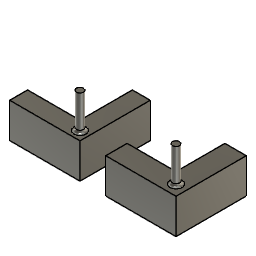
Laser+L_s (Autodesk Fusion 360 design; units mm, degrees)
Autodesk Fusion 360 part; units mm, degrees
note: some values were not read from the file. Set by a fixed rule: which sketch regions a step uses.
sketch "Sketch1" plane through (0, 0, 0) normal (0, 0, 1) x (1, 0, 0)
  line L0 (0, 0) -> (20.5, 0)
  line L1 (20.5, 0) -> (20.5, 80.5)
  line L2 (20.5, 80.5) -> (0, 80.5)
  line L3 (0, 80.5) -> (0, 0)
  line L4 (0, 0) -> (-60, 0)
  line L5 (-60, 0) -> (-60, 20.5)
  line L6 (-60, 20.5) -> (0, 20.5)
  line L7 (0, 20.5) -> (0, 0)
  dimension "d1" = 20.5
  dimension "d2" = 60
  dimension "d3" = 20.5
  dimension "d4" = 80.5
  constraint horizontal L0
  constraint vertical L1
  constraint horizontal L2
  constraint vertical L3
  constraint coincident L0.start L3.end
  constraint horizontal L4
  constraint vertical L5
  constraint horizontal L6
  constraint vertical L7
  measures "d1" distance of L0.start L0.end
  measures "d2" distance of L5.end L6.end
  measures "d3" distance of L4.end L5.end
  measures "d4" distance of L0.end L1.end
extrude "Extrude1" add sketch "Sketch1" along normal blind 40 makes body 1
sketch "Sketch3" plane through (0, 0, 0) normal (0, 0, -1) x (1, 0, 0)
  line L0 (20.5, 0) -> (-60, 0)
  line L1 (-60, 0) -> (-60, -20.5)
  line L2 (-60, -20.5) -> (0, -20.5)
  line L3 (0, -20.5) -> (0, -80.5)
  line L4 (0, -80.5) -> (20.5, -80.5)
  line L5 (20.5, -80.5) -> (20.5, 0)
  line L6 (14.0377, -6.3471) -> (0.9042, -6.3471) construction
  line L7 (0.9042, -6.3471) -> (0.9042, -16.8864) construction
  line L8 (0.9042, -16.8864) -> (14.0377, -16.8864) construction
  line L9 (14.0377, -16.8864) -> (14.0377, -6.3471) construction
  dimension "d7" = 12
  text T0 "R" font "Arial" height 12 align left top in box 13.1336 x 10.5393 at (14.0377, -6.3471) x (-1, 0) y (0, -1) spacing 1
extrude "Extrude2" cut sketch "Sketch3" against normal blind 3 text T0 bodies 1
sketch "Sketch4" plane through (0, 0, 40) normal (0, 0, 1) x (-1, 0, 0)
  line L0 (60, 0) -> (-20.5, 0)
  line L1 (-20.5, 0) -> (-20.5, -80.5)
  line L2 (-20.5, -80.5) -> (0, -80.5)
  line L3 (0, -80.5) -> (0, -20.5)
  line L4 (0, -20.5) -> (60, -20.5)
  line L5 (60, -20.5) -> (60, 0)
  line L6 (0, -20.5) -> (-20.5, 0)
  circle A0 centre (-10.25, -10.25) radius 4
  dimension "d10" = 8
  constraint coincident L3.end L4.start
  constraint coincident L0.end L1.start
  constraint midpoint L6 A0.centre
  measures "d10" diameter of A0
extrude "Extrude3" add sketch "Sketch4" along normal blind 40 contours L6 A0 | L6 A0 bodies 1
fillet "Fillet1" radius 3 1 edges at (13.9793, 8.8035, 40) on bodies 1
sketch "Sketch5" plane through (0, 0, 0) normal (0, 0, 1) x (1, 0, 0)
  line L0 (50, 0) -> (130.5, 0)
  line L1 (130.5, 0) -> (130.5, 24.5)
  line L2 (130.5, 24.5) -> (50, 24.5)
  line L3 (50, 24.5) -> (50, 0)
  line L4 (130.5, 0) -> (106, 0)
  line L5 (106, 0) -> (106, 80.5)
  line L6 (106, 80.5) -> (130.5, 80.5)
  line L7 (130.5, 80.5) -> (130.5, 0)
  dimension "d15" = 24.5
  dimension "d16" = 80.5
  dimension "d17" = 24.5
  dimension "d18" = 80.5
  constraint horizontal L0
  constraint vertical L1
  constraint horizontal L2
  constraint vertical L3
  constraint horizontal L4
  constraint vertical L5
  constraint horizontal L6
  constraint vertical L7
  measures "d15" distance of L0.start L2.end
  measures "d16" distance of L0.start L0.end
  measures "d17" distance of L0.end L4.end
  measures "d18" distance of L0.end L6.end
extrude "Extrude4" add sketch "Sketch5" along normal blind 40 separate body makes body 2
sketch "Sketch6" plane through (0, 0, 0) normal (0, 0, -1) x (1, 0, 0)
  line L0 (50, -24.5) -> (106, -24.5)
  line L1 (106, -24.5) -> (106, -80.5)
  line L2 (106, -80.5) -> (130.5, -80.5)
  line L3 (130.5, -80.5) -> (130.5, 0)
  line L4 (130.5, 0) -> (50, 0)
  line L5 (50, 0) -> (50, -24.5)
  line L6 (120.6614, -6.2816) -> (105.6614, -6.2816) construction
  line L7 (105.6614, -6.2816) -> (105.6614, -21.2816) construction
  line L8 (105.6614, -21.2816) -> (120.6614, -21.2816) construction
  line L9 (120.6614, -21.2816) -> (120.6614, -6.2816) construction
  dimension "d21" = 12
  text T0 "L" font "Arial" height 12 align left top in box 15 x 15 at (120.6614, -6.2816) x (-1, 0) y (0, -1) spacing 1
extrude "Extrude5" cut sketch "Sketch6" against normal blind 3 text T0 bodies 2
sketch "Sketch7" plane through (0, 0, 40) normal (0, 0, 1) x (-1, 0, 0)
  line L0 (-106, -24.5) -> (-50, -24.5)
  line L1 (-50, -24.5) -> (-50, 0)
  line L2 (-50, 0) -> (-130.5, 0)
  line L3 (-130.5, 0) -> (-130.5, -80.5)
  line L4 (-130.5, -80.5) -> (-106, -80.5)
  line L5 (-106, -80.5) -> (-106, -24.5)
  line L6 (-106, -24.5) -> (-130.5, 0)
  circle A0 centre (-118.25, -12.25) radius 4
  dimension "d24" = 8
  constraint coincident L0.start L5.end
  constraint coincident L2.end L3.start
  constraint midpoint L6 A0.centre
  measures "d24" diameter of A0
extrude "Extrude6" add sketch "Sketch7" along normal blind 40 contours L6 A0 | L6 A0 bodies 2
fillet "Fillet2" radius 3 1 edges at (121.9793, 10.8035, 40) on bodies 2
equation "d4 = 60 mm + 20.5 mm"
